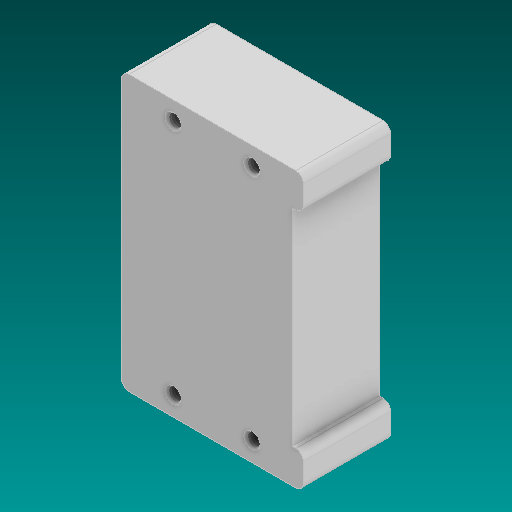
# Autodesk Inventor part: hoefijzer
Saved by Autodesk Inventor 2020.2 (Build 242310000, 310)
## iProperties
Created: 2020-05-19
Part Number: hoefijzer
Material: Generic
Document SubType Name: Modeling
Designer: Svend
Density: 1 g/cm^3
Appearance: Default
Author: Svend
Autodesk Inventor part; units mm, degrees
ref_plane "YZ Plane" through (0, 0, 0) normal (1, 0, 0) x (0, 1, 0)
ref_plane "XZ Plane" through (0, 0, 0) normal (0, 1, 0) x (-1, 0, 0)
ref_plane "Work Plane1" through (0, 0, 0) normal (0, 0, 1) x (1, 0, 0)
sketch "Sketch1" plane through (0, 0, 0) normal (0, 0, 1) x (1, 0, 0)
  line L0 (-42.2638, -6.6778) -> (-4.2638, -6.6778) projected
  line L1 (-44.2638, -77.1778) -> (-44.2638, -8.6778) projected
  line L2 (-4.2638, -79.1778) -> (-42.2638, -79.1778) projected
  line L3 (-2.2638, -8.6778) -> (-2.2638, -77.1778) projected
  circle A0 centre (-23.2638, -42.9278) radius 12.6 projected
  circle A1 centre (-7.2638, -42.9278) radius 2 projected
  circle A2 centre (-23.2638, -58.9278) radius 2 projected
  circle A3 centre (-11.9501, -54.2415) radius 1.5 projected
  circle A4 centre (-34.5775, -54.2415) radius 1.5 projected
  circle A5 centre (-11.9501, -31.6141) radius 1.5 projected
  circle A6 centre (-23.2638, -26.9278) radius 2 projected
  circle A7 centre (-34.5775, -31.6141) radius 1.5 projected
  circle A8 centre (-39.2638, -42.9278) radius 2 projected
  arc A9 (-38.6638, -72.0778) -> (-38.6638, -76.2778) centre (-38.6638, -74.1778) ccw projected
  line L4 (-7.8638, -72.0778) -> (-38.6638, -72.0778) projected
  arc A10 (-7.8638, -76.2778) -> (-7.8638, -72.0778) centre (-7.8638, -74.1778) ccw projected
  line L5 (-38.6638, -76.2778) -> (-7.8638, -76.2778) projected
  arc A11 (-7.8638, -13.7778) -> (-7.8638, -9.5778) centre (-7.8638, -11.6778) ccw projected
  line L6 (-38.6638, -13.7778) -> (-7.8638, -13.7778) projected
  arc A12 (-38.6638, -9.5778) -> (-38.6638, -13.7778) centre (-38.6638, -11.6778) ccw projected
  line L7 (-7.8638, -9.5778) -> (-38.6638, -9.5778) projected
  line L8 (30.6247, -21.3479) -> (-25.1038, -35.8635) projected
  arc A13 (-25.1038, -35.8635) -> (-25.1038, -49.9921) centre (-23.2638, -42.9278) ccw projected
  line L9 (-25.1038, -49.9921) -> (30.6247, -64.5078) projected
  arc A14 (30.6247, -64.5078) -> (30.6247, -21.3479) centre (36.2457, -42.9278) ccw projected
  arc A15 (-24.9022, -36.6377) -> (-24.9022, -49.2179) centre (-23.2638, -42.9278) ccw projected
  line L10 (30.8264, -22.122) -> (-24.9022, -36.6377) projected
  arc A16 (30.8264, -63.7336) -> (30.8264, -22.122) centre (36.2457, -42.9278) ccw projected
  line L11 (-24.9022, -49.2179) -> (30.8264, -63.7336) projected
  line L12 (-44.2638, -15.6778) -> (-2.2638, -15.6778)
  line L13 (-2.2638, -70.1778) -> (-44.2638, -70.1778)
  line L14 (-35.2638, -68.1778) -> (-35.2638, -17.6778)
  line L15 (-47.2638, -8.6778) -> (-47.2638, -77.1778)
  line L16 (-45.2638, -6.6778) -> (-4.2638, -6.6778)
  line L17 (-45.2638, -79.1778) -> (-4.2638, -79.1778)
  arc A17 (-45.2638, -6.6778) -> (-47.2638, -8.6778) centre (-45.2638, -8.6778) ccw
  arc A18 (-47.2638, -77.1778) -> (-45.2638, -79.1778) centre (-45.2638, -77.1778) ccw
  arc A19 (-33.2638, -15.6778) -> (-35.2638, -17.6778) centre (-33.2638, -17.6778) ccw
  arc A20 (-35.2638, -68.1778) -> (-33.2638, -70.1778) centre (-33.2638, -68.1778) ccw
  line L18 (0.7362, -72.1778) -> (0.7362, -77.1778)
  line L19 (0.7362, -8.6778) -> (0.7362, -13.6778)
  line L20 (-2.2638, -15.6778) -> (-1.2638, -15.6778)
  line L21 (-4.2638, -6.6778) -> (-1.2638, -6.6778)
  line L22 (-2.2638, -70.1778) -> (-1.2638, -70.1778)
  line L23 (-4.2638, -79.1778) -> (-1.2638, -79.1778)
  arc A21 (0.7362, -8.6778) -> (-1.2638, -6.6778) centre (-1.2638, -8.6778) ccw
  arc A22 (-1.2638, -15.6778) -> (0.7362, -13.6778) centre (-1.2638, -13.6778) ccw
  arc A23 (0.7362, -72.1778) -> (-1.2638, -70.1778) centre (-1.2638, -72.1778) ccw
  arc A24 (-1.2638, -79.1778) -> (0.7362, -77.1778) centre (-1.2638, -77.1778) ccw
  line L24 (-44.2638, -70.1778) -> (-44.2638, -15.6778)
  arc A25 (-2.2638, -8.6778) -> (-4.2638, -6.6778) centre (-4.2638, -8.6778) ccw projected
  arc A26 (-42.2638, -6.6778) -> (-44.2638, -8.6778) centre (-42.2638, -8.6778) ccw projected
  arc A27 (-44.2638, -77.1778) -> (-42.2638, -79.1778) centre (-42.2638, -77.1778) ccw projected
  arc A28 (-4.2638, -79.1778) -> (-2.2638, -77.1778) centre (-4.2638, -77.1778) ccw projected
  point P0 (0, 0)
  point P1 (-35.2638, -15.6778)
  point P2 (-35.2638, -70.1778)
  point P3 (-12.8638, -11.6778)
  point P4 (-33.6638, -11.6778)
  point P5 (-33.6638, -74.1778)
  point P6 (-12.8638, -74.1778)
  point P7 (-35.2638, -55.5753)
  point P8 (-35.2638, -52.9077)
  point P9 (-35.2638, -46.7697)
  point P10 (-35.2638, -39.0859)
  point P11 (-35.2638, -32.9479)
  point P12 (-35.2638, -30.2803)
  point P13 (-47.2638, -6.6778)
  point P14 (-47.2638, -79.1778)
  point P15 (0.7362, -70.1778)
  point P16 (0.7362, -79.1778)
  point P17 (0.7362, -6.6778)
  point P18 (0.7362, -15.6778)
  point P19 (-42.2638, -6.6778)
  dimension "d0" = 9
  dimension "d1" = 9
  dimension "d2" = 9
  dimension "d3" = 5
  dimension "d4" = 5
  dimension "d5" = 5
  dimension "d6" = 5
  dimension "d9" = 3
  dimension "d12" = 3
  dimension "d13" = 3
  constraints: 26 end point, 24 point on line, 16 point on circle, 16 tangent, 12 horizontal alignment, 8 centre point, 5 equal radius, 4 collinear, 3 horizontal, 3 vertical
  measures "d0" distance between parallel lines of L1 L14
  measures "d1" distance between parallel lines of L2 L13
  measures "d2" distance between parallel lines of L0 L12
  measures "d3" distance of point (-33.664, -11.678) A12.centre
  measures "d4" distance of A11.centre point (-12.864, -11.678)
  measures "d5" distance of A10.centre point (-12.864, -74.178)
  measures "d6" distance of A9.centre point (-33.664, -74.178)
  measures "d9" distance between parallel lines of L15 L1
  measures "d12" distance between parallel lines of L18 L3
  measures "d13" distance between parallel lines of L19 L3
extrude "Extrusion1" add sketch "Sketch1" along normal blind 23 contours A26 L1 A27 L17 A18 L15 A17 L16 | L0 A25 L3 L12 L1 A26 | L21 A21 L19 A22 L20 L3 A25 | L12 A19 L14 A7 A0 A4 A20 L13 L1 | L3 L8 A5 A0 L14 A7 A19 L12 | L13 L3 A28 L2 A27 L1 | L3 L10 A0 L8 A5 | A20 L14 A4 A0 L9 A3 L3 L13 | L3 L11 A0 L10 | L8 A5 | A5 L8 | L22 A23 L18 A24 L23 A28 L3 | L14 A7 | A7 L14 | L3 L9 A3 A0 L11 | L10 A15 L11 A0 L9 A13 L8 | A0 L11 A15 L10 | L14 A4 | A4 L14 | L8 A13 L9 A0 L14 | L9 A3 | A3 L9 | L14 A0 | A1 | A2 | A6 | A8 | L4 A10 L5 A9 | L6 A12 L7 A11
sketch "Sketch2" plane through (0, 0, 23) normal (0, 0, 1) x (1, 0, 0)
  arc A0 (-1.2638, -15.6778) -> (0.7362, -13.6778) centre (-1.2638, -13.6778) ccw projected
  line L0 (0.7362, -13.6778) -> (0.7362, -8.6778) projected
  arc A1 (0.7362, -8.6778) -> (-1.2638, -6.6778) centre (-1.2638, -8.6778) ccw projected
  arc A2 (-45.2638, -6.6778) -> (-47.2638, -8.6778) centre (-45.2638, -8.6778) ccw projected
  line L1 (-47.2638, -8.6778) -> (-47.2638, -77.1778) projected
  arc A3 (-47.2638, -77.1778) -> (-45.2638, -79.1778) centre (-45.2638, -77.1778) ccw projected
  arc A4 (-1.2638, -79.1778) -> (0.7362, -77.1778) centre (-1.2638, -77.1778) ccw projected
  line L2 (0.7362, -77.1778) -> (0.7362, -72.1778) projected
  arc A5 (0.7362, -72.1778) -> (-1.2638, -70.1778) centre (-1.2638, -72.1778) ccw projected
  line L3 (-1.2638, -70.1778) -> (-2.2638, -70.1778) projected
  line L4 (-2.2638, -15.6778) -> (-1.2638, -15.6778) projected
  line L5 (-2.2638, -70.1778) -> (-2.2638, -15.6778) projected
  line L6 (-1.2638, -6.6778) -> (-45.2638, -6.6778) projected
  line L7 (-45.2638, -79.1778) -> (-1.2638, -79.1778) projected
  point P0 (0, 0)
  point P1 (-12.8638, -11.6778)
  point P2 (-33.6638, -11.6778)
  point P3 (-33.6638, -74.1778)
  point P4 (-12.8638, -74.1778)
hole "Hole1" at (-12.8638, -11.6778, 23) at (-33.6638, -11.6778, 23) at (-33.6638, -74.1778, 23) at (-12.8638, -74.1778, 23) direction (0, 0, -1) diameter 3.242 end through all thread size "M4x0.7" class "6H" standard "ISO Metric profile"
chamfer "Chamfer1" distance 0.5 angle 45 8 edges at (-33.6638, -72.5568, 23) (-12.8638, -72.5568, 23) (-33.6638, -10.0568, 23) (-12.8638, -10.0568, 23) (-33.6638, -72.5568, 0) (-12.8638, -72.5568, 0) (-33.6638, -10.0568, 0) (-12.8638, -10.0568, 0)
equation "\"d1\" = d2"
equation "\"d2\" = d0"
equation "\"d4\" = d3"
equation "\"d5\" = d4"
equation "\"d6\" = d5"
equation "\"d12\" = d9"
equation "\"d13\" = d12"
body "Solid1"
